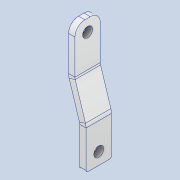
# Autodesk Inventor part: ForearmActuatorConnector2
Saved by Autodesk Inventor 2020 (Build 240168000, 168)
## iProperties
Created: 2020-04-15
Part Number: ForearmActuatorConnector2
Material: Aluminum 6061
Document SubType Name: Sheet Metal
Designer: valer
Density: 2.7 g/cm^3
Sheet Metal Rule: Default
Appearance: Aluminum - Flat
Author: valer
Autodesk Inventor part; units mm, degrees
ref_plane "YZ Plane" through (0, 0, 0) normal (1, 0, 0) x (0, 1, 0)
ref_plane "XZ Plane" through (0, 0, 0) normal (0, 1, 0) x (-1, 0, 0)
ref_plane "XY Plane" through (0, 0, 0) normal (0, 0, 1) x (1, 0, 0)
sketch "Base" plane through (0, 0, 0) normal (0, 0, 1) x (1, 0, 0)
  line L0 (0, 19.05) -> (0, -3.81)
  line L1 (5.588, -21.59) -> (5.588, -41.95)
  line L2 (0, 13.05) -> (2.54, 13.05) construction
  line L3 (2.54, 13.05) -> (2.54, 8.05) construction
  line L4 (2.54, 8.05) -> (0, 8.05) construction
  line L5 (0, 8.05) -> (0, 13.05)
  line L6 (8.128, -30.95) -> (5.588, -30.95) construction
  line L7 (5.588, -30.95) -> (5.588, -35.95) construction
  line L8 (5.588, -35.95) -> (8.128, -35.95) construction
  line L9 (8.128, -35.95) -> (8.128, -30.95) construction
  line L10 (0, 10.55) -> (38.6405, 10.55) construction
  line L11 (5.588, -33.45) -> (38.6405, -33.45) construction
  line L12 (38.6405, -33.45) -> (38.6405, 10.55) construction
  line L13 (5.588, -21.59) -> (0, -3.81)
  dimension "d39" = 5
  dimension "d41" = 6
  dimension "d42" = 2.54
  dimension "d43" = 6
  dimension "d44" = 44
  dimension "d60" = 5.588
  dimension "d61" = 17.78
  dimension "d62" = 22.86
  measures "d39" distance of L2.end L3.end
  measures "d41" distance from line of L0.start L2
  measures "d42" distance of L2.start L2.end
  measures "d43" distance from line of L1.end L8
  measures "d44" distance of L11.end L10.end
  measures "d60" distance between parallel lines of L0 L1
  measures "d61" vertical distance of L1.start L0.end
  measures "d62" distance of L0.end L0.start
contour flange "BaseFeature" sketch "Base" thickness 3.17 bend radius 3.17 width 12.7 along (0, 0, 1) mid plane no both sides no wall seen from (0, 7.62, 0) lies toward (-1, 0, 0) curves L0 L13 L1
bend "Bend1"
corner "Corner1"
fillet "FilletsFeature" radius 5 2 edges at (-1.585, 19.05, 12.7) (-1.585, 19.05, 0)
sketch "ForearmHole" plane through (0, -11.6974, 12.7) normal (1, 0, 0) x (0, 0, -1)
  circle A0 centre (6.35, 24.7474) radius 2.5
  line L0 (7.7, 30.7474) -> (5, 30.7474) construction
  line L1 (6.35, 30.7474) -> (6.35, 24.7474) construction
  dimension "d45" = 5
  dimension "d63" = 6
  constraints: 2 end point, 1 centre point, 1 midpoint, 1 vertical
  measures "d45" diameter of A0
  measures "d63" distance of L1.start L1.end
hole "ForearmHoleFeature" at (0, 13.05, 6.35) direction (-1, 0, 0) diameter 5 end through all
sketch "ActuatorMountHole" plane through (5.588, -19.9053, 12.7) normal (1, 0, 0) x (0, 0, -1)
  circle A0 centre (6.35, -16.0447) radius 2.5
  line L0 (12.7, -22.0447) -> (0, -22.0447) projected
  line L1 (6.35, -16.0447) -> (6.35, -22.0447) construction
  line L2 (12.7, -22.0447) -> (0, -22.0447) projected
  dimension "d47" = 5
  dimension "d48" = 6
  constraints: 2 end point, 1 centre point, 1 midpoint, 1 perpendicular
  measures "d47" diameter of A0
  measures "d48" distance from line of L0 L1.start
hole "ActuatorMountHoleFeature" at (5.588, -35.95, 6.35) direction (-1, 0, 0) diameter 5 end through all
fillet "EndFilletsFeature" radius 1 2 edges at (4.003, -41.95, 12.7) (4.003, -41.95, 0)
equation "\"d43\" = d41"
equation "\"d63\" = d41"
equation "\"d17\" = Thickness"
equation "\"d48\" = d41"
equation "\"d36\" = Thickness"
equation "\"d0\" = Thickness"
equation "\"d1\" = BendReliefWidth"
equation "\"d2\" = BendReliefDepth"
equation "\"d3\" = MinimumRemnant"
equation "\"d4\" = TransitionRadius"
equation "\"d6\" = BendRadius"
equation "\"d8\" = CornerReliefSize"
equation "\"d9\" = GapSize"
equation "\"d10\" = JacobiRadiusSize"
equation "\"BendRadius\" = Thickness"
equation "\"BendReliefWidth\" = Thickness"
equation "\"BendReliefDepth\" = 0.5 * Thickness"
equation "\"CornerReliefSize\" = 4 * Thickness"
equation "\"MinimumRemnant\" = 2 * Thickness"
equation "\"TransitionRadius\" = BendRadius"
equation "\"JacobiRadiusSize\" = BendRadius"
equation "\"GapSize\" = Thickness"
equation "\"Thickness\" = 3.17"
body "Solid1"
